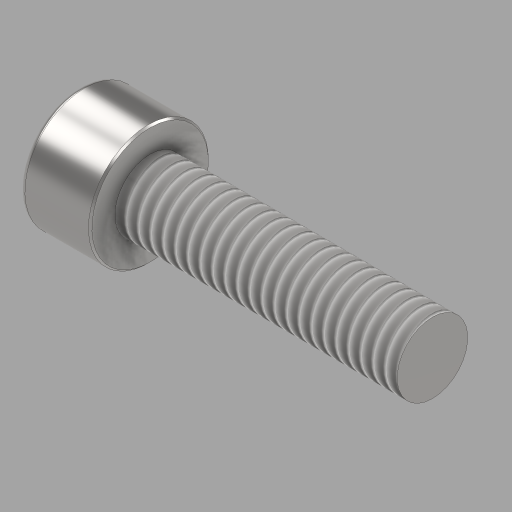
# Autodesk Inventor part: Screw_StainlessSteal_M4_SocketCap_20mm
Saved by Autodesk Inventor 2024 (Build 280153020, 153B)
## iProperties
Created: 2022-02-03
Part Number: Screw_StainlessSteal_M4_SocketCap_20mm
Material: Stainless Steel
Document SubType Name: Modeling
Designer: schanen
Density: 8 g/cm^3
Appearance: Semi-Polished
Author: schanen
Autodesk Inventor part; units mm, degrees
ref_plane "YZ Plane" through (0, 0, 0) normal (1, 0, 0) x (0, 1, 0)
ref_plane "XZ Plane" through (0, 0, 0) normal (0, 1, 0) x (-1, 0, 0)
ref_plane "XY Plane" through (0, 0, 0) normal (0, 0, 1) x (1, 0, 0)
sketch "Sketch1" plane through (0, 0, 0) normal (0, 0, 1) x (1, 0, 0)
  line L0 (0, 0) -> (-20, 0)
  line L1 (-20, 0) -> (-20, 3.4)
  line L2 (-20, 3.4) -> (-16, 3.4)
  line L3 (-16, 3.4) -> (-16, 2)
  line L4 (-16, 2) -> (0, 2)
  line L5 (0, 2) -> (0, 0)
  dimension "d0" = 4
  dimension "d1" = 2
  dimension "d2" = 20
  dimension "d3" = 3.4
  constraints: 12 end point, 5 perpendicular, 1 horizontal
  measures "d0" distance of L1.end L2.end
  measures "d1" distance between parallel lines of L0 L4
  measures "d2" distance of L0.start L0.end
  measures "d3" distance of L0.end L1.end
revolve "Revolution1" add sketch "Sketch1" angle 360 about axis through (0, 0, 0) along (-1, 0, 0)
fillet "Fillet1" radius 0.3 1 edges at (-20, -3.4, 0)
chamfer "Chamfer1" distance 0.1 angle 45 1 edges at (-16, -3.4, 0)
thread "Thread1" size "M4x0.7" class "6g" standard "ANSI Metric M Profile" full length
sketch "Sketch2" plane through (-20, 0, 0) normal (-1, 0, 0) x (0, 0, 1)
  line L0 (-1.1237, 1.3558) -> (0.6123, 1.651)
  line L1 (0.6123, 1.651) -> (1.736, 0.2952)
  line L2 (1.736, 0.2952) -> (1.1237, -1.3558)
  line L3 (1.1237, -1.3558) -> (-0.6123, -1.651)
  line L4 (-0.6123, -1.651) -> (-1.736, -0.2952)
  line L5 (-1.736, -0.2952) -> (-1.1237, 1.3558)
  point P0 (0, 0)
  point P1 (0, 0)
  dimension "d11" = 3.05
  constraints: 12 end point, 1 coincident, 13 other
  measures "d11" distance between parallel lines of L4 L1
extrude "Extrusion1" cut sketch "Sketch2" against normal blind 2.5
body "Solid1"
